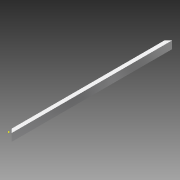
# Autodesk Inventor part: 42in 2x1 boxbeam
Saved by Autodesk Inventor 2015 (Build 190159000, 159)
## iProperties
Created: 2015-01-11
Part Number: 42in 2x1 boxbeam
Material: Generic
Document SubType Name: Modeling
Designer: chapale16
Density: 1 g/cm^3
Appearance: Chrome - Polished
Author: chapale16
Autodesk Inventor part; units mm, degrees
ref_plane "YZ Plane" through (0, 0, 0) normal (1, 0, 0) x (0, 1, 0)
ref_plane "XZ Plane" through (0, 0, 0) normal (0, 1, 0) x (-1, 0, 0)
ref_plane "XY Plane" through (0, 0, 0) normal (0, 0, 1) x (1, 0, 0)
sketch "Sketch2" plane through (0, 0, 0) normal (0, 0, 1) x (1, 0, 0)
  line L0 (-4.1078, 5.9023) -> (21.2922, 5.9023)
  line L1 (21.2922, 5.9023) -> (21.2922, -44.8977)
  line L2 (21.2922, -44.8977) -> (-4.1078, -44.8977)
  line L3 (-4.1078, -44.8977) -> (-4.1078, 5.9023)
  line L4 (18.1934, 2.8035) -> (-1.009, 2.8035)
  line L5 (-1.009, 2.8035) -> (-1.009, -41.7989)
  line L6 (-1.009, -41.7989) -> (18.1934, -41.7989)
  line L7 (18.1934, -41.7989) -> (18.1934, 2.8035)
  point P0 (0, 0)
  dimension "d0" = 25.4
  dimension "d1" = 50.8
  dimension "d2" = 3.0988
  constraints: 16 end point, 4 parallel, 2 perpendicular, 1 horizontal, 3 other
  measures "d0" distance of L1.end L2.end
  measures "d1" distance of L0.end L1.end
  measures "d2" distance between parallel lines of L0 L4
extrude "Extrusion1" add sketch "Sketch2" along normal blind 1066.8
sketch "Sketch5" plane through (0, 0, 1066.8) normal (0, 0, 1) x (1, 0, 0)
  point P0 (0, 0)
sketch "Sketch6" plane through (-4.1078, 5.9023, 0) normal (0, 1, 0) x (1, 0, 0)
  line L0 (25.4, 0) -> (-1.2066, -26.6066)
  line L1 (0, 0) -> (0, -1066.8) projected
  line L2 (0, -25.4) -> (0, 0)
  line L3 (0, 0) -> (25.4, 0)
  line L4 (0, -1066.8) -> (25.4, -1066.8) projected
  line L5 (25.4, -1066.8) -> (-7.0638, -1034.3362)
  line L6 (25.4, -1066.8) -> (71.3108, -1066.8) construction
  line L7 (0, -1041.4) -> (0, -1066.8)
  line L8 (0, -1066.8) -> (25.4, -1066.8)
  point P0 (4.1078, 0)
  dimension "d11" = 135
  constraints: 14 end point, 4 point on line, 2 perpendicular, 1 collinear, 1 equal length, 1 horizontal, 1 vertical
  measures "d11" angle of L6 L5
extrude "Extrusion2" cut sketch "Sketch6" against normal blind 1066.8 contours L0 L1 L3
extrude "Extrusion3" cut sketch "Sketch6" against normal blind 1066.8 contours L5 L4 L1
body "Solid1"
